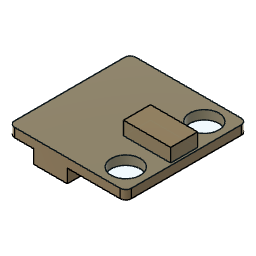
PulseOximeterClip (Autodesk Fusion 360 archive; units mm, degrees)
design "gy-MAX30102"
Autodesk Fusion 360 part; units mm, degrees
sketch "Sketch1" plane through (0, 0, 0) normal (0, 0, 1) x (1, 0, 0)
  line L0 (0, 0) -> (13.716, 0)
  line L1 (13.716, 0) -> (13.716, 13.208)
  line L2 (13.716, 13.208) -> (0, 13.208)
  line L3 (0, 13.208) -> (0, 0)
  dimension "d1" = 13.716
  dimension "d2" = 13.208
  constraint horizontal L0
  constraint vertical L1
  constraint horizontal L2
  constraint vertical L3
  constraint coincident L0.start L3.end
  measures "d1" distance of L0.start L0.end
  measures "d2" distance of L0.start L2.end
extrude "Extrude1" add sketch "Sketch1" along normal blind 1.016
fillet "Fillet1" radius 0.635 4 edges at (13.716, 0, 0.508) (13.716, 13.208, 0.508) (0, 0, 0.508) (0, 13.208, 0.508)
sketch "Sketch2" plane through (0, 0, 1.016) normal (0, 0, 1) x (-1, 0, 0)
  arc A0 (-0.635, -13.208) -> (0, -12.573) centre (-0.635, -12.573) ccw
  line L0 (0, -12.573) -> (0, -0.635)
  arc A1 (0, -0.635) -> (-0.635, 0) centre (-0.635, -0.635) ccw
  line L1 (-0.635, 0) -> (-13.081, 0)
  arc A2 (-13.081, 0) -> (-13.716, -0.635) centre (-13.081, -0.635) ccw
  line L2 (-13.716, -0.635) -> (-13.716, -12.573)
  arc A3 (-13.716, -12.573) -> (-13.081, -13.208) centre (-13.081, -12.573) ccw
  line L3 (-13.081, -13.208) -> (-0.635, -13.208)
  line L4 (-13.716, -2.8777) -> (0, -2.8777)
  line L5 (0, -2.8777) -> (0, -5.08)
  line L6 (0, -5.08) -> (-13.716, -5.08)
  line L7 (-13.716, -5.08) -> (-13.716, -2.8777)
  line L8 (-13.716, -5.4805) -> (0, -5.4805)
  line L9 (0, -5.4805) -> (0, -9.2905)
  line L10 (0, -9.2905) -> (-13.716, -9.2905)
  line L11 (-13.716, -9.2905) -> (-13.716, -5.4805)
  dimension "d9" = 13.716
  dimension "d10" = 3.81
  constraint horizontal L4
  constraint vertical L5
  constraint horizontal L6
  constraint vertical L7
  constraint coincident L0 L5.end
  constraint coincident L2 L4.start
  constraint horizontal L8
  constraint vertical L9
  constraint horizontal L10
  constraint vertical L11
  constraint coincident L2 L8.start
  measures "d9" distance of L8.start L8.end
  measures "d10" distance of L8.start L10.end
extrude "Extrude4" add sketch "Sketch2" along normal blind 1.524 contours L0 L2 L8 L9 L10 L11
sketch "Sketch3" plane through (0, 0, 0) normal (0, 0, -1) x (1, 0, 0)
  arc A0 (0, -12.573) -> (0.635, -13.208) centre (0.635, -12.573) ccw
  line L0 (0.635, -13.208) -> (13.081, -13.208)
  arc A1 (13.081, -13.208) -> (13.716, -12.573) centre (13.081, -12.573) ccw
  line L1 (13.716, -12.573) -> (13.716, -0.635)
  arc A2 (13.716, -0.635) -> (13.081, 0) centre (13.081, -0.635) ccw
  line L2 (13.081, 0) -> (0.635, 0)
  arc A3 (0.635, 0) -> (0, -0.635) centre (0.635, -0.635) ccw
  line L3 (0, -0.635) -> (0, -12.573)
  line L4 (6.858, 0) -> (8.382, 0)
  line L5 (8.382, -0.254) -> (8.382, -5.334)
  line L6 (6.858, 0) -> (5.334, 0)
  line L7 (5.334, -0.254) -> (5.334, -5.334)
  line L8 (8.382, -0.254) -> (5.334, -0.254)
  line L9 (5.334, -0.254) -> (5.334, -5.588)
  line L10 (5.334, -5.588) -> (8.382, -5.588)
  line L11 (8.382, -5.588) -> (8.382, -0.254)
  dimension "d15" = 1.524
  dimension "d19" = 0.254
  dimension "d20" = 5.334
  constraint horizontal L4
  constraint vertical L5
  constraint midpoint L2 L4.start
  constraint horizontal L6
  constraint vertical L7
  constraint horizontal L8
  constraint vertical L9
  constraint horizontal L10
  constraint vertical L11
  measures "d15" distance of L4.start L4.end
  measures "d19" distance of L4.end L5.start
  measures "d20" distance of L5.start L10.end
extrude "Extrude5" add sketch "Sketch3" along normal blind 1.27 contours A0 L0 A1 L1 A2 L2 A3 L3 L4 L6 | L5 L7 L8 L9 L10 L11
extrude "Extrude7" cut 1 faces at (8.9323, 8.8053, -1.27) along direction (0, 0, 1) blind 1.27
extrude "Extrude8" add sketch "Sketch3" along normal blind 0.254
extrude "Extrude9" add sketch "Sketch3" along normal blind 1.778 contours L5 L7 L8 L9 L10 L11
extrude "Extrude10" cut 2 faces at (8.9323, 10.5963, 1.016) (4.7837, 3.6537, 1.016) along direction (0, 0, -1) blind 0.254
extrude "Extrude11" cut 1 faces at (4.572, 8.0205, 2.54) along direction (0, 0, -1) blind 0.254
extrude "Extrude12" cut 1 faces at (4.572, 8.0205, 2.286) along direction (0, 0, -1) blind 1.524
sketch "Sketch4" plane through (0, 0, 0.762) normal (0, 0, 1) x (-1, 0, 0)
  line L0 (-13.716, -0.635) -> (-13.716, -12.573)
  arc A0 (-13.716, -12.573) -> (-13.081, -13.208) centre (-13.081, -12.573) ccw
  line L1 (-13.081, -13.208) -> (-0.635, -13.208)
  arc A1 (-0.635, -13.208) -> (0, -12.573) centre (-0.635, -12.573) ccw
  line L2 (0, -12.573) -> (0, -0.635)
  arc A2 (0, -0.635) -> (-0.635, 0) centre (-0.635, -0.635) ccw
  line L3 (-0.635, 0) -> (-13.081, 0)
  arc A3 (-13.081, 0) -> (-13.716, -0.635) centre (-13.081, -0.635) ccw
  line L4 (-6.858, 0) -> (-6.858, -6.604) construction
  line L5 (-6.858, -6.604) -> (0, -6.604)
  line L6 (0, -6.604) -> (0, -10.414)
  line L7 (0, -10.414) -> (-6.858, -10.414)
  line L8 (-6.858, -6.604) -> (-13.716, -6.604)
  line L9 (-13.716, -6.604) -> (-13.716, -10.4252)
  line L10 (-13.716, -10.4252) -> (-6.858, -10.4252)
  line L11 (-6.858, -10.4252) -> (-6.858, -10.414)
  dimension "d35" = 6.604
  dimension "d36" = 3.81
  dimension "d37" = 3.8212
  constraint midpoint L3 L4.start
  constraint perpendicular L3 L4
  constraint horizontal L5
  constraint vertical L6
  constraint horizontal L7
  constraint horizontal L8
  constraint vertical L9
  constraint horizontal L10
  constraint vertical L11
  constraint coincident L0 L9.end
  measures "d35" distance of L4.start L4.end
  measures "d36" distance of L4.end L7.end
  measures "d37" distance of L4.end L10.end
extrude "Extrude13" add sketch "Sketch4" along normal blind 1.524 contours L0 L2 L5 L6 L7 L8 L9 L10 L11
sketch "Sketch5" plane through (0, 0, 0.762) normal (0, 0, 1) x (-1, 0, 0)
  line L0 (-6.858, 0) -> (-6.858, -3.556) construction
  line L1 (-6.858, -3.556) -> (-7.62, -3.556)
  line L2 (-7.62, -3.556) -> (-7.62, -4.064)
  line L3 (-7.62, -4.064) -> (-6.858, -4.064)
  line L4 (-6.858, -3.556) -> (-6.096, -3.556)
  line L5 (-6.096, -3.556) -> (-6.096, -4.064)
  line L6 (-6.096, -4.064) -> (-6.858, -4.064)
  point P0 (-6.858, 0)
  dimension "d40" = 3.556
  dimension "d41" = 0.762
  dimension "d42" = 0.508
  dimension "d43" = 0.508
  constraint coincident P0 L0.start
  constraint horizontal L1
  constraint vertical L2
  constraint horizontal L3
  constraint horizontal L4
  constraint vertical L5
  constraint horizontal L6
  measures "d40" distance of P0 L0.end
  measures "d41" distance of L0.end L1.end
  measures "d42" distance of L0.end L3.end
  measures "d43" distance of L0.end L3.end
extrude "Extrude14" add sketch "Sketch5" along normal blind 1.016
sketch "Sketch6" plane through (0, 0, -0.254) normal (0, 0, -1) x (1, 0, 0)
  line L0 (8.382, -0.254) -> (8.382, -5.588)
  line L1 (8.382, -5.588) -> (5.334, -5.588)
  line L2 (5.334, -5.588) -> (5.334, -0.254)
  line L3 (5.334, -0.254) -> (8.382, -0.254)
  line L4 (13.081, 0) -> (0.635, 0)
  arc A0 (0.635, 0) -> (0, -0.635) centre (0.635, -0.635) ccw
  line L5 (0, -0.635) -> (0, -12.573)
  arc A1 (0, -12.573) -> (0.635, -13.208) centre (0.635, -12.573) ccw
  line L6 (0.635, -13.208) -> (13.081, -13.208)
  arc A2 (13.081, -13.208) -> (13.716, -12.573) centre (13.081, -12.573) ccw
  line L7 (13.716, -12.573) -> (13.716, -0.635)
  arc A3 (13.716, -0.635) -> (13.081, 0) centre (13.081, -0.635) ccw
  line L8 (2.413, -0.762) -> (2.413, -2.413)
  line L9 (0, -2.413) -> (2.413, -2.413)
  circle A4 centre (2.413, -2.413) radius 1.651
  line L10 (11.43, 0) -> (11.43, -2.413)
  line L11 (13.716, -2.413) -> (11.303, -2.413)
  circle A5 centre (11.303, -2.413) radius 1.651
  dimension "d47" = 2.413
  dimension "d48" = 3.302
  dimension "d49" = 2.413
  dimension "d50" = 2.413
  dimension "d51" = 3.302
  constraint vertical L8
  constraint coincident L5 L9.start
  constraint perpendicular L8 L9
  constraint coincident L8.end L9.end
  constraint coincident A4 L8.start
  constraint coincident L4 L10.start
  constraint perpendicular L4 L10
  constraint coincident L7 L11.start
  constraint perpendicular L10 L11
  constraint coincident L11.end A5.centre
  measures "d47" distance of L9.start L8.end
  measures "d48" diameter of A4
  measures "d49" distance of L10.start L10.end
  measures "d50" distance of L11.start L11.end
  measures "d51" diameter of A5
extrude "Extrude15" cut sketch "Sketch6" against normal blind 1.524 contours L10 L11 A5 | L10 L11 A5 | L8 L9 A4 | L8 L9 A4
sketch "Sketch7" plane through (0, 0, 0.762) normal (0, 0, 1) x (-1, 0, 0)
  line L0 (-6.858, -10.4252) -> (-13.716, -10.4252)
  line L1 (-13.716, -10.4252) -> (-13.716, -12.573)
  arc A0 (-13.716, -12.573) -> (-13.081, -13.208) centre (-13.081, -12.573) ccw
  line L2 (-13.081, -13.208) -> (-0.635, -13.208)
  arc A1 (-0.635, -13.208) -> (0, -12.573) centre (-0.635, -12.573) ccw
  line L3 (0, -12.573) -> (0, -10.414)
  line L4 (0, -10.414) -> (-6.858, -10.414)
  line L5 (-6.858, -10.414) -> (-6.858, -10.4252)
  line L6 (-6.858, -10.414) -> (-6.858, -10.922)
  dimension "d54" = 0.508
  constraint coincident L4.end L5.start
  constraint perpendicular L0 L6
  measures "d54" distance of L4.end L6.end
sketch "Sketch8" plane through (0, 0, -0.254) normal (0, 0, -1) x (1, 0, 0)
  circle A0 centre (11.303, -2.413) radius 1.651
  circle A1 centre (2.413, -2.413) radius 1.651
  line L0 (8.382, -0.254) -> (8.382, -5.588)
  line L1 (8.382, -5.588) -> (5.334, -5.588)
  line L2 (5.334, -5.588) -> (5.334, -0.254)
  line L3 (5.334, -0.254) -> (8.382, -0.254)
  line L4 (13.081, 0) -> (0.635, 0)
  arc A2 (0.635, 0) -> (0, -0.635) centre (0.635, -0.635) ccw
  line L5 (0, -0.635) -> (0, -12.573)
  arc A3 (0, -12.573) -> (0.635, -13.208) centre (0.635, -12.573) ccw
  line L6 (0.635, -13.208) -> (13.081, -13.208)
  arc A4 (13.081, -13.208) -> (13.716, -12.573) centre (13.081, -12.573) ccw
  line L7 (13.716, -12.573) -> (13.716, -0.635)
  arc A5 (13.716, -0.635) -> (13.081, 0) centre (13.081, -0.635) ccw
extrude "Extrude6" [suppressed]
extrude "Extrude3" [suppressed]
equation "d21 = 0,05 in + 0,06 in"
equation "d47 = 0,03 in + 0,065 in"
equation "d49 = 0,03 in + 0,065 in"
